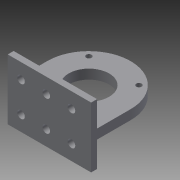
# Autodesk Inventor part: ff12_mount
Saved by Autodesk Inventor 2014 (Build 180170000, 170)
## iProperties
Created: 2014-08-22
Part Number: ff12_mount
Material: Generic
Document SubType Name: Modeling
Designer: Matthew
Density: 1 g/cm^3
Appearance: Default
Author: Matthew
Autodesk Inventor part; units mm, degrees
ref_plane "YZ Plane" through (0, 0, 0) normal (1, 0, 0) x (0, 1, 0)
ref_plane "XZ Plane" through (0, 0, 0) normal (0, 1, 0) x (-1, 0, 0)
ref_plane "XY Plane" through (0, 0, 0) normal (0, 0, 1) x (1, 0, 0)
sketch "Sketch1" plane through (0, 0, 0) normal (0, 0, 1) x (1, 0, 0)
  circle A0 centre (0, 0) radius 17
  arc A1 (35, 0) -> (-35, 0) centre (0, 0) ccw
  line L0 (-35, 0) -> (-35, -28.1305)
  line L1 (-35, -28.1305) -> (35, -28.1305)
  line L2 (35, -28.1305) -> (35, 0)
  circle A2 centre (-21, 21) radius 2.25
  circle A3 centre (21, 21) radius 2.25
  circle A4 centre (-21, -21) radius 2.25
  circle A5 centre (21, -21) radius 2.25
  dimension "d0" = 34
  dimension "d1" = 70
  dimension "d2" = 70
  dimension "d3" = 28.1305
  dimension "d54" = 4.5
  dimension "d57" = 42
  dimension "d60" = 42
  dimension "d63" = 21
  dimension "d64" = 21
  constraints: 6 centre point, 6 end point, 2 coincident, 2 point on circle, 2 tangent, 2 vertical, 1 horizontal, 1 perpendicular, 6 other
  measures "d0" diameter of A0
  measures "d1" diameter of A1
  measures "d2" distance of L0.end L1.end
  measures "d3" distance of L1.end L2.end
  measures "d54" diameter of A2
  measures "d57" distance of A2.centre A3.centre
  measures "d60" distance of A2.centre A4.centre
  measures "d63" horizontal distance of point (0, 0) A4.centre
  measures "d64" horizontal distance of A2.centre point (0, 0)
extrude "Extrusion1" add sketch "Sketch1" along normal blind 8 contours L2 L1 L0 A1 | A2 | A3 | A4 | A5
sketch "Sketch2" plane through (-35, -28.1305, 0) normal (0, -1, 0) x (1, 0, 0)
  line L0 (0, 0) -> (70, 0) construction
  line L1 (0, 0) -> (0, 8) projected
  line L2 (0, -21.4) -> (70, -21.4)
  line L3 (70, -21.4) -> (70, 29.4)
  line L4 (70, 29.4) -> (0, 29.4)
  line L5 (0, 29.4) -> (0, -21.4)
  line L6 (0, -21.4) -> (70, 29.4) construction
  line L7 (70, -21.4) -> (0, 29.4) construction
  point P0 (35, 0)
  point P1 (35, 4)
  point P2 (35, 4)
  point P3 (0, 4)
  point P4 (35, 4)
  point P5 (35, 0)
  point P6 (70, 8)
  dimension "d7" = 50.8
  dimension "d65" = 70
  dimension "d66" = 70
  constraints: 12 end point, 6 midpoint, 2 parallel, 1 horizontal, 1 horizontal alignment, 1 perpendicular, 1 vertical alignment
  measures "d7" distance of L2.end L3.end
  measures "d65" distance of L3.end L4.end
  measures "d66" distance of L1.end point (70, 8)
extrude "Extrusion2" add sketch "Sketch2" along normal blind 5
sketch "Sketch3" plane through (-35, -33.1305, 0) normal (0, -1, 0) x (1, 0, 0)
  line L0 (70, 29.4) -> (0, 29.4) projected
  line L1 (0, 29.4) -> (0, -21.4) projected
  point P0 (35, 0)
  point P1 (11.1875, 16.7)
  point P2 (32.3542, 16.7)
  point P3 (11.1875, -8.7)
  point P4 (32.3542, -8.7)
  point P5 (53.5208, 16.7)
  point P6 (53.5208, -8.7)
  dimension "d39" = 21.1667
  dimension "d42" = 25.4
  dimension "d45" = 12.7
  dimension "d67" = 70
  dimension "d68" = 50.8
  dimension "d70" = 11.1875
  constraints: 1 horizontal, 1 vertical, 5 other
  measures "d39" distance of point (11.187, 16.7) point (32.354, 16.7)
  measures "d42" distance of point (11.187, 16.7) point (11.187, -8.7)
  measures "d45" distance from line of L0 point (11.187, 16.7)
  measures "d67" distance of L0.start L0.end
  measures "d68" distance of L0.end L1.end
  measures "d70" distance from line of L1 point (11.187, 16.7)
hole "Hole2" at (-23.8125, -33.1305, 16.7) at (-2.6458, -33.1305, 16.7) at (-23.8125, -33.1305, -8.7) at (-2.6458, -33.1305, -8.7) at (18.5208, -33.1305, 16.7) at (18.5208, -33.1305, -8.7) direction (0, 1, 0) diameter 6.35 end through all
sketch "Sketch4" plane through (0, 0, 0) normal (0, 0, -1) x (-1, 0, 0)
  circle A0 centre (0, 0) radius 17 projected
  line L0 (35, 0) -> (35, -28.1305) projected
  line L1 (35, -28.1305) -> (-35, -28.1305) projected
  point P0 (-21, 21)
  point P1 (21, 21)
  point P2 (-21, -21)
  point P3 (21, -21)
  dimension "d80" = 42
  dimension "d83" = 42
  dimension "d86" = 21
  dimension "d87" = 21
  constraints: 1 horizontal, 1 vertical, 3 other
  measures "d80" distance of point (-21, 21) point (21, 21)
  measures "d83" distance of point (-21, 21) point (-21, -21)
  measures "d86" horizontal distance of A0.centre point (-21, 21)
  measures "d87" horizontal distance of point (-21, 21) A0.centre
hole "Hole3" at (21, 21, 0) at (-21, 21, 0) at (21, -21, 0) at (-21, -21, 0) direction (0, 0, 1) diameter 4.5 end through all
equation "\"d2\" = d1"
equation "\"d63\" = 0.5 * d60"
equation "\"d64\" = d63"
equation "\"d65\" = d66"
equation "\"d70\" = -0.5 * d69 + 0.5 * d67"
equation "\"d83\" = d80"
equation "\"d86\" = 0.5 * d80"
equation "\"d87\" = d86"
equation "\"d69\" = 47.625"
body "Solid1"
